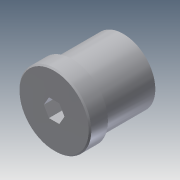
# Autodesk Inventor part: Colson Hub
Saved by Autodesk Inventor 2014 SP1 (Build 180222100, 222)
## iProperties
Created: 2013-11-29
Part Number: Colson Hub
Material: Aluminum 6061
Document SubType Name: Modeling
Designer: Rauhul Varma
Mass: 141.784 g
Surface Area: 101.23 cm^2
Volume: 52.3188 cm^3
Density: 2.71 g/cm^3
Appearance: Aluminum - Flat
Author: Rauhul Varma
Autodesk Inventor part; units mm, degrees
ref_plane "YZ Plane" through (0, 0, 0) normal (1, 0, 0) x (0, 1, 0)
ref_plane "XZ Plane" through (0, 0, 0) normal (0, 1, 0) x (-1, 0, 0)
ref_plane "XY Plane" through (0, 0, 0) normal (0, 0, 1) x (1, 0, 0)
sketch "Sketch1" plane through (0, 0, 0) normal (0, 0, 1) x (1, 0, 0)
  circle A0 centre (0, 0) radius 11.1125
  dimension "d0" = 22.225
  constraints: 1 centre point, 1 coincident
  measures "d0" diameter of A0
extrude "Bearing Offset" add sketch "Sketch1" along normal blind 1.5875
sketch "Sketch2" plane through (0, 0, 1.5875) normal (0, 0, 1) x (1, 0, 0)
  circle A0 centre (0, 0) radius 11.1125 projected
  circle A1 centre (0, 0) radius 19.8438
  dimension "d3" = 39.6875
  constraints: 1 centre point, 1 coincident
  measures "d3" diameter of A1
extrude "Colson Hub (Press Fit)" add sketch "Sketch2" along normal blind 31.75 contours A0 | A1
sketch "Sketch3" plane through (0, 0, 33.3375) normal (0, 0, 1) x (1, 0, 0)
  circle A0 centre (0, 0) radius 19.8438 projected
  circle A1 centre (0, 0) radius 22.225
  dimension "d6" = 44.45
  constraints: 1 centre point, 1 coincident
  measures "d6" diameter of A1
extrude "Colson Retension" add sketch "Sketch3" along normal blind 11.1125 contours A0 | A1
sketch "Sketch4" plane through (0, 0, 0) normal (0, 0, -1) x (-1, 0, 0)
  circle A0 centre (0, 0) radius 11.1125 projected
  line L0 (3.2079, 5.5563) -> (6.4158, 0)
  line L1 (6.4158, 0) -> (3.2079, -5.5563)
  line L2 (3.2079, -5.5563) -> (-3.2079, -5.5563)
  line L3 (-3.2079, -5.5563) -> (-6.4158, 0)
  line L4 (-6.4158, 0) -> (-3.2079, 5.5563)
  line L5 (-3.2079, 5.5563) -> (3.2079, 5.5563)
  dimension "d9" = 11.1125
  constraints: 12 end point, 1 coincident, 1 horizontal, 13 other
  measures "d9" distance between parallel lines of L2 L5
extrude "7/16\" Hex" cut sketch "Sketch4" against normal through all contours L0 L1 L2 L3 L4 L5
chamfer "End Chamfers" distance 0.7937 angle 45 2 edges at (-11.1125, 0, 0) (-22.225, 0, 44.45)
body "Solid1"
